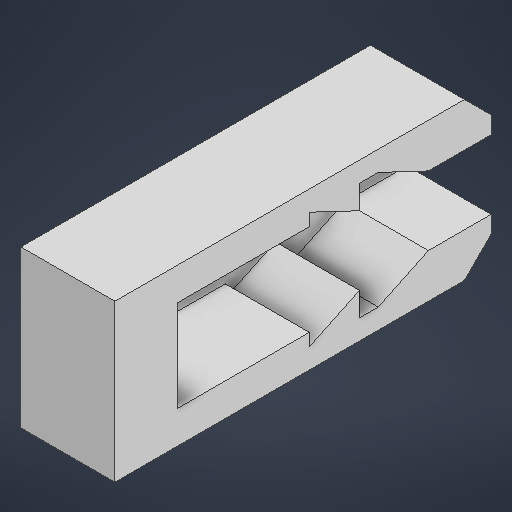
# Autodesk Inventor part: встав для крюка
Saved by Autodesk Inventor 2025 (Build 290162000, 162)
## iProperties
Created: 2025-02-20
Part Number: встав для крюка
Material: Типовые
Document SubType Name: Modeling
Designer: Phantom
Density: 1 g/cm^3
Appearance: По умолчанию
Author: Phantom
Autodesk Inventor part; units mm, degrees
ref_plane "YZ Plane" through (0, 0, 0) normal (1, 0, 0) x (0, 1, 0)
ref_plane "XZ Plane" through (0, 0, 0) normal (0, 1, 0) x (-1, 0, 0)
ref_plane "XY Plane" through (0, 0, 0) normal (0, 0, 1) x (1, 0, 0)
sketch "Эскиз1" plane through (0, 0, 0) normal (0, 1, 0) x (-1, 0, 0)
  line L0 (0, 0) -> (22, 0)
  line L1 (22, 0) -> (22, 60)
  line L2 (22, 60) -> (0, 60)
  line L3 (0, 60) -> (0, 0)
  dimension "d0" = 22
  dimension "d1" = 60
  constraints: 8 end point, 2 parallel, 1 horizontal, 1 perpendicular
  measures "d0" distance of L2.end L1.end
  measures "d1" distance of L1.end L0.end
extrude "Выдавливание1" add sketch "Эскиз1" along normal blind 25
sketch "Эскиз2" plane through (0, 0, 60) normal (1, 0, 0) x (0, 0, -1)
  line L0 (60, 25) -> (0, 25) projected
  line L1 (60, 25) -> (60, 21.8)
  line L2 (60, 0) -> (60, 25) projected
  line L3 (60, 21.8) -> (20, 21.8)
  line L4 (60, 0) -> (0, 0) projected
  line L5 (60, 0) -> (60, 3.2)
  line L6 (60, 3.2) -> (20, 3.2)
  line L7 (20, 25) -> (20, 0)
  line L8 (20, 21.8) -> (28, 21.8)
  line L9 (20, 12.5) -> (60, 12.5)
  line L10 (60, 12.5) -> (60, 18)
  line L11 (60, 18) -> (13, 18)
  line L12 (28, 21.8) -> (28, 18)
  line L13 (28, 18) -> (20, 21.8)
  line L14 (28, 21.8) -> (31, 21.8)
  line L15 (31, 21.8) -> (39, 21.8)
  line L16 (39, 21.8) -> (39, 18)
  line L17 (39, 18) -> (31, 21.8)
  line L18 (39, 21.8) -> (42, 21.8)
  line L19 (42, 21.8) -> (50, 21.8)
  line L20 (50, 21.8) -> (50, 18)
  line L21 (42, 21.8) -> (50, 18)
  line L22 (20, 3.2) -> (28, 3.2)
  line L23 (28, 3.2) -> (28, 7)
  line L24 (28, 7) -> (20, 3.2)
  line L25 (31, 3.2) -> (39, 3.2)
  line L26 (39, 3.2) -> (39, 7)
  line L27 (39, 7) -> (31, 3.2)
  line L28 (42, 3.2) -> (50, 3.2)
  line L29 (50, 3.2) -> (50, 7)
  line L30 (42, 3.2) -> (50, 7)
  line L31 (50, 7) -> (63, 7)
  point P0 (22, 21.8)
  point P1 (60, 7)
  dimension "d4" = 3.2
  dimension "d5" = 3.2
  dimension "d6" = 40
  dimension "d7" = 5.5
  dimension "d8" = 8
  dimension "d9" = 8
  dimension "d10" = 3
  dimension "d11" = 8
  constraints: 58 end point, 15 point on line, 8 symmetric about line, 5 perpendicular, 2 midpoint, 1 horizontal, 1 parallel, 1 vertical
  measures "d4" distance of L0.start L1.end
  measures "d5" distance of L2.start L5.end
  measures "d6" distance between parallel lines of L2 L7
  measures "d7" distance of L9.end L10.end
  measures "d8" distance of L3.end L8.end
  measures "d9" distance of L14.end L15.end
  measures "d10" distance of L15.end L18.end
  measures "d11" distance of L18.end L19.end
extrude "Выдавливание2" cut sketch "Эскиз2" against normal through all contours L13 L11 L7 | L2 L9 L7 L11 | L3 L17 L11 L12 | L2 L31 L30 L6 L26 L27 L23 L24 L7 L9 | L11 L16 L3 L21
sketch "Эскиз3" plane through (0, 0, 60) normal (1, 0, 0) x (0, 0, -1)
  line L0 (50, 18) -> (60, 18) projected
  line L1 (60, 18) -> (60, 25) projected
  line L2 (0, 25) -> (60, 25) projected
  line L3 (0, 0) -> (0, 25) projected
  line L4 (0, 0) -> (60, 0) projected
  line L5 (60, 0) -> (60, 7) projected
  line L6 (60, 7) -> (50, 7) projected
  line L7 (50, 7) -> (42, 3.2) projected
  line L8 (42, 3.2) -> (39, 3.2) projected
  line L9 (39, 3.2) -> (39, 7) projected
  line L10 (39, 7) -> (31, 3.2) projected
  line L11 (31, 3.2) -> (28, 3.2) projected
  line L12 (28, 3.2) -> (28, 7) projected
  line L13 (28, 7) -> (20, 3.2) projected
  line L14 (20, 3.2) -> (20, 21.8) projected
  line L15 (20, 21.8) -> (28, 18) projected
  line L16 (28, 18) -> (28, 21.8) projected
  line L17 (28, 21.8) -> (31, 21.8) projected
  line L18 (31, 21.8) -> (39, 18) projected
  line L19 (39, 18) -> (39, 21.8) projected
  line L20 (39, 21.8) -> (42, 21.8) projected
  line L21 (42, 21.8) -> (50, 18) projected
chamfer "Фаска1" distance 4.25 angle 45 2 edges at (-11, 0, 0) (-11, 25, 0)
sketch "Эскиз4" plane through (0, 0, 60) normal (1, 0, 0) x (0, 0, -1)
  line L0 (20, 21.8) -> (28, 18) projected
  line L1 (20, 21.8) -> (31, 21.8)
  line L2 (31, 21.8) -> (31, 16.575)
  line L3 (31, 16.575) -> (20, 16.575)
  line L4 (20, 16.575) -> (20, 21.8)
  line L5 (20, 3.2) -> (20, 21.8) projected
  line L6 (20, 3.2) -> (30, 3.2)
  line L7 (30, 3.2) -> (30, 12)
  line L8 (30, 12) -> (20, 12)
  line L9 (20, 12) -> (20, 3.2)
  line L10 (20, 21.8) -> (10, 21.8)
  line L11 (10, 21.8) -> (10, 3.2)
  line L12 (10, 3.2) -> (20, 3.2)
  line L13 (20, 3.2) -> (20, 21.8)
  point P0 (60, 0)
  constraints: 24 end point, 6 parallel, 3 horizontal, 3 perpendicular
extrude "Выдавливание3" cut sketch "Эскиз4" against normal through all
sketch "Эскиз5" plane through (0, 0, 60) normal (1, 0, 0) x (0, 0, -1)
  line L0 (31, 3.2) -> (10, 3.2) projected
  line L1 (10, 3.2) -> (10, 21.8) projected
  line L2 (10, 21.8) -> (31, 21.8) projected
  line L3 (31, 21.8) -> (39, 18) projected
  line L4 (39, 18) -> (39, 21.8) projected
  line L5 (39, 21.8) -> (42, 21.8) projected
  line L6 (42, 21.8) -> (50, 18) projected
  line L7 (50, 18) -> (60, 18) projected
  line L8 (60, 18) -> (60, 20.75) projected
  line L9 (55.75, 25) -> (60, 20.75) projected
  line L10 (0, 25) -> (55.75, 25) projected
  line L11 (0, 0) -> (0, 25) projected
  line L12 (0, 0) -> (55.75, 0) projected
  line L13 (60, 4.25) -> (55.75, 0) projected
  line L14 (60, 4.25) -> (60, 7) projected
  line L15 (60, 7) -> (50, 7) projected
  line L16 (50, 7) -> (42, 3.2) projected
  line L17 (42, 3.2) -> (39, 3.2) projected
  line L18 (39, 3.2) -> (39, 7) projected
  line L19 (39, 7) -> (31, 3.2) projected
  point P0 (60, 0)
extrude "Выдавливание4" cut sketch "Эскиз5" against normal blind 7
sketch "Эскиз6" plane through (-22, 0, 60) normal (-1, 0, 0) x (0, 0, 1)
  line L0 (-10, 21.8) -> (-10, 3.2) projected
  line L1 (-10, 3.2) -> (-10, 5.2)
  line L2 (-10, 5.2) -> (-31, 5.2)
  line L3 (-31, 5.2) -> (-31, 3.2)
  line L4 (-10, 3.2) -> (-31, 3.2) projected
  line L5 (-31, 3.2) -> (-39, 7) projected
  line L6 (-39, 7) -> (-39, 3.2) projected
  line L7 (-39, 3.2) -> (-42, 3.2) projected
  line L8 (-42, 3.2) -> (-50, 7) projected
  line L9 (-50, 7) -> (-60, 7) projected
  line L10 (-60, 4.25) -> (-60, 7) projected
  line L11 (-55.75, 0) -> (-60, 4.25) projected
  line L12 (-55.75, 0) -> (0, 0) projected
  line L13 (0, 0) -> (0, 25) projected
  line L14 (-55.75, 25) -> (0, 25) projected
  line L15 (-60, 20.75) -> (-55.75, 25) projected
  line L16 (-60, 18) -> (-60, 20.75) projected
  line L17 (-60, 18) -> (-50, 18) projected
  line L18 (-50, 18) -> (-42, 21.8) projected
  line L19 (-42, 21.8) -> (-39, 21.8) projected
  line L20 (-39, 21.8) -> (-39, 18) projected
  line L21 (-39, 18) -> (-31, 21.8) projected
  line L22 (-31, 21.8) -> (-10, 21.8) projected
  line L23 (-10, 21.8) -> (-10, 3.2) projected
  line L24 (-10, 21.8) -> (-31, 21.8)
  line L25 (-31, 21.8) -> (-31, 19.8)
  line L26 (-31, 19.8) -> (-10, 19.8)
  line L27 (-10, 19.8) -> (-10, 21.8)
  point P0 (-60, 0)
  point P1 (-31, 3.2)
  point P2 (-31, 21.8)
  dimension "d21" = 2
  dimension "d22" = 21
  dimension "d23" = 2
  constraints: 14 end point, 3 perpendicular, 2 parallel, 1 horizontal, 1 point on line
  measures "d21" distance of L0.end L1.end
  measures "d22" distance of L26.end L25.end
  measures "d23" distance of L25.end L24.end
extrude "Выдавливание5" add sketch "Эскиз6" against normal up to surface (15 mm away) contours L0 L26 L25 L22 | L0 L4 L3 L2
sketch "Эскиз7" plane through (-22, 0, 60) normal (-1, 0, 0) x (0, 0, 1)
  line L0 (-10, 19.8) -> (-10, 5.2) projected
  line L1 (-10, 5.2) -> (-25, 5.2)
  line L2 (-25, 5.2) -> (-25, 9.2)
  line L3 (-25, 9.2) -> (-10, 9.2)
  line L4 (-10, 9.2) -> (-10, 5.2)
  line L5 (-10, 19.8) -> (-25, 19.8)
  line L6 (-25, 19.8) -> (-25, 15.8)
  line L7 (-25, 15.8) -> (-10, 15.8)
  line L8 (-10, 15.8) -> (-10, 19.8)
  line L9 (-31, 3.2) -> (-39, 7) projected
  line L10 (-39, 7) -> (-39, 3.2) projected
  line L11 (-39, 3.2) -> (-42, 3.2) projected
  line L12 (-42, 3.2) -> (-50, 7) projected
  line L13 (-50, 7) -> (-60, 7) projected
  line L14 (-60, 4.25) -> (-60, 7) projected
  line L15 (-55.75, 0) -> (-60, 4.25) projected
  line L16 (-55.75, 0) -> (0, 0) projected
  line L17 (0, 0) -> (0, 25) projected
  line L18 (-55.75, 25) -> (0, 25) projected
  line L19 (-60, 20.75) -> (-55.75, 25) projected
  line L20 (-60, 18) -> (-60, 20.75) projected
  line L21 (-60, 18) -> (-50, 18) projected
  line L22 (-50, 18) -> (-42, 21.8) projected
  line L23 (-42, 21.8) -> (-39, 21.8) projected
  line L24 (-39, 21.8) -> (-39, 18) projected
  line L25 (-39, 18) -> (-31, 21.8) projected
  line L26 (-31, 21.8) -> (-31, 19.8) projected
  line L27 (-31, 19.8) -> (-10, 19.8) projected
  line L28 (-10, 19.8) -> (-10, 5.2) projected
  line L29 (-10, 5.2) -> (-31, 5.2) projected
  line L30 (-31, 5.2) -> (-31, 3.2) projected
  line L31 (-60, 18) -> (-60, 7)
  line L32 (-25, 9.2) -> (-60, 9.2)
  line L33 (-25, 15.8) -> (-64.95, 15.8)
  line L34 (-30.4379, 9.2) -> (-10, 5.2)
  line L35 (-30.4379, 15.8) -> (-10, 19.8)
  point P0 (-60, 0)
  point P1 (-25, 19.8)
  point P2 (-25, 5.2)
  point P3 (-25, 5.2)
  point P4 (-60, 15.8)
  point P5 (-25, 19.8)
  dimension "d27" = 4
  dimension "d29" = 4
  constraints: 26 end point, 4 parallel, 3 horizontal, 3 perpendicular, 3 point on line, 1 vertical
  measures "d27" distance of L1.end L2.end
  measures "d29" distance of L6.end L5.end
extrude "Выдавливание6" add sketch "Эскиз7" against normal blind 1.6 contours L35 L6 L5 | L6 L35 L33 L31 L21 L22 L23 L24 L25 L26 L27 | L1 L2 L34 | L29 L30 L9 L10 L11 L12 L13 L31 L32 L34 L2
